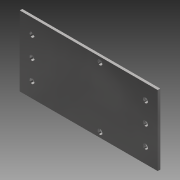
# Autodesk Inventor part: Part77
Saved by Autodesk Inventor 2015 (Build 190159000, 159)
## iProperties
Created: 2015-01-11
Part Number: Part77
Material: Generic
Document SubType Name: Modeling
Designer: mastkee16
Density: 1 g/cm^3
Appearance: Knurled 45
Author: mastkee16
Autodesk Inventor part; units mm, degrees
ref_plane "YZ Plane" through (0, 0, 0) normal (1, 0, 0) x (0, 1, 0)
ref_plane "XZ Plane" through (0, 0, 0) normal (0, 1, 0) x (-1, 0, 0)
ref_plane "XY Plane" through (0, 0, 0) normal (0, 0, 1) x (1, 0, 0)
sketch "Sketch1" plane through (0, 0, 0) normal (0, 0, 1) x (1, 0, 0)
  line L0 (0, 0) -> (174.7774, 0)
  line L1 (174.7774, 0) -> (174.7774, 88.9)
  line L2 (174.7774, 88.9) -> (0, 88.9)
  line L3 (0, 88.9) -> (0, 0)
  dimension "d0" = 174.7774
  dimension "d1" = 88.9
  constraints: 8 end point, 2 parallel, 1 horizontal, 1 perpendicular
  measures "d0" distance of L2.end L1.end
  measures "d1" distance of L1.end L0.end
extrude "Extrusion1" add sketch "Sketch1" along normal blind 3.175
sketch "Sketch2" plane through (0, 0, 3.175) normal (0, 0, 1) x (1, 0, 0)
  line L0 (174.7774, 88.9) -> (0, 88.9) projected
  line L1 (0, 0) -> (174.7774, 0) projected
  line L2 (174.7774, 0) -> (174.7774, 88.9) projected
  line L3 (0, 88.9) -> (0, 0) projected
  point P0 (15.5321, 69.85)
  point P1 (159.2453, 69.85)
  point P2 (15.5321, 44.45)
  point P3 (159.2453, 44.45)
  point P4 (159.2453, 19.05)
  point P5 (15.5321, 19.05)
  dimension "d6" = 88.9
  dimension "d9" = 15.5321
  dimension "d12" = 15.5321
  dimension "d31" = 25.4
  dimension "d32" = 25.4
  dimension "d33" = 25.4
  dimension "d34" = 25.4
  dimension "d35" = 69.85
  dimension "d36" = 69.85
  dimension "d37" = 143.7132
  measures "d6" distance between parallel lines of L1 L0
  measures "d9" distance from line of L2 point (159.245, 69.85)
  measures "d12" distance from line of L3 point (15.532, 69.85)
  measures "d31" distance of point (15.532, 44.45) point (15.532, 69.85)
  measures "d32" distance of point (159.245, 44.45) point (159.245, 69.85)
  measures "d33" distance of point (159.245, 19.05) point (159.245, 44.45)
  measures "d34" distance of point (15.532, 19.05) point (15.532, 44.45)
  measures "d35" distance from line of L1 point (159.245, 69.85)
  measures "d36" distance from line of L1 point (15.532, 69.85)
  measures "d37" distance of point (159.245, 69.85) point (15.532, 69.85)
hole "Hole1" at (15.5321, 69.85, 3.175) at (159.2453, 69.85, 3.175) at (15.5321, 44.45, 3.175) at (15.5321, 19.05, 3.175) at (159.2453, 19.05, 3.175) at (159.2453, 44.45, 3.175) direction (0, 0, -1) diameter 6.35 end through all
sketch "Sketch3" plane through (0, 0, 3.175) normal (0, 0, 1) x (1, 0, 0)
  line L0 (0, 88.9) -> (0, 0) projected
  line L1 (174.7774, 88.9) -> (0, 88.9) projected
  line L2 (0, 0) -> (174.7774, 0) projected
  point P0 (101.5873, 82.55)
  point P1 (101.5873, 6.35)
  dimension "d20" = 101.5873
  dimension "d21" = 101.5873
  dimension "d22" = 6.35
  dimension "d23" = 6.35
  measures "d20" distance from line of point (101.587, 82.55) L0
  measures "d21" distance from line of point (101.587, 6.35) L0
  measures "d22" distance from line of L1 point (101.587, 82.55)
  measures "d23" distance from line of L2 point (101.587, 6.35)
hole "Hole2" at (101.5873, 82.55, 3.175) at (101.5873, 6.35, 3.175) direction (0, 0, -1) diameter 6.35 end through all
body "Solid1"
